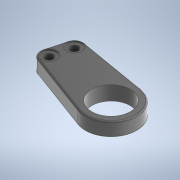
# Autodesk Inventor part: RearBumper
Saved by Autodesk Inventor 2020.4 (Build 244396000, 396)
## iProperties
Created: 2022-01-16
Part Number: RearBumper
Material: PC/ABS プラスチック
Document SubType Name: Modeling
Designer: Masato Kubotera
Density: 0.357273 g/cm^3
Appearance: 滑らか - 黒
Author: Masato Kubotera
Autodesk Inventor part; units mm, degrees
ref_plane "YZ Plane" through (0, 0, 0) normal (1, 0, 0) x (0, 1, 0)
ref_plane "XZ Plane" through (0, 0, 0) normal (0, 1, 0) x (-1, 0, 0)
ref_plane "XY Plane" through (0, 0, 0) normal (0, 0, 1) x (1, 0, 0)
derived "Trunk_basis.ipt"
sketch "スケッチ1" plane through (0, 0, 0) normal (0, 1, 0) x (-1, 0, 0)
  line L0 (0, 22) -> (0, -142.9) construction
  circle A0 centre (5, 0) radius 10.5 construction
  line L1 (-7, 16) -> (36, 16) construction
  line L2 (36, 16) -> (36, -16) construction
  line L3 (36, -16) -> (-7, -16) construction
  line L4 (-7, -16) -> (-7, 16) construction
  line L5 (-7, 16) -> (36, -16) construction
  line L6 (36, 16) -> (-7, -16) construction
  line L7 (33, 13.5) -> (6, 13.5) construction
  line L8 (6, 13.5) -> (6, -13.5) construction
  line L9 (6, -13.5) -> (33, -13.5) construction
  line L10 (33, -13.5) -> (33, 13.5) construction
  line L11 (33, 13.5) -> (6, -13.5) construction
  line L12 (6, 13.5) -> (33, -13.5) construction
  line L13 (-7, 0) -> (36, 0) construction
  arc A1 (5, 16) -> (-7, 10.583) centre (5, 0) ccw construction
  line L14 (34.5651, -16.05) -> (5, -16.05)
  line L15 (5, 16.05) -> (34.5651, 16.05)
  line L16 (36.05, 14.5651) -> (36.05, -14.5651)
  line L17 (36.05, -16.05) -> (-7.05, 16.05) construction
  line L18 (-7.05, -16.05) -> (36.05, 16.05) construction
  arc A2 (5, 16.05) -> (-6.5314, 11.1638) centre (5, 0) ccw
  arc A3 (-6.5314, 11.1638) -> (-7.05, 9.8372) centre (-6.0721, 10.2196) ccw
  arc A4 (36.05, 14.5651) -> (34.5651, 16.05) centre (35.3075, 15.3075) ccw
  circle A5 centre (6, 13.5) radius 1.35
  line L19 (19.5, 13.5) -> (19.5, -13.5) construction
  circle A6 centre (33, 13.5) radius 1.35
  line L20 (-12, 22) -> (-17, 17)
  line L21 (-17, 17) -> (-17, -16)
  line L22 (-17, -16) -> (-28.5, -27.5)
  line L23 (-28.5, -27.5) -> (-28.5, -103)
  line L24 (54.5, -22.5) -> (54.5, 17)
  line L25 (54.5, 17) -> (49.5, 22)
  line L26 (49.5, 22) -> (-12, 22)
  line L27 (-35.5597, -116.5529) -> (-28.5, -142.9)
  line L28 (-16, -139) -> (-16, -94) construction
  line L29 (-7.5, -140.4849) -> (-7.5, -142.9)
  line L30 (-7.5, -142.9) -> (7.5, -142.9)
  line L31 (7.5, -140.4849) -> (7.5, -142.9)
  arc A7 (-7.5, -140.4849) -> (-8.9849, -139) centre (-8.2425, -139.7425) ccw
  line L32 (-17.5, -138.9955) -> (-17.5, -133) construction
  line L33 (-19, -133) -> (-16, -133) construction
  line L34 (-19, -133) -> (-19, -139) construction
  line L35 (-16, -133) -> (-16, -139) construction
  line L36 (-12, 22) -> (-7, 22) construction
  line L37 (-7, 22) -> (-7, -22) construction
  line L38 (-7, -22) -> (-12, -22) construction
  line L39 (-12, -22) -> (-12, 22) construction
  line L40 (-12, 22) -> (-7, -22) construction
  line L41 (-7, 22) -> (-12, -22) construction
  line L42 (-9.5, 22) -> (-9.5, -22) construction
  line L43 (-7, 0) -> (-12, 0) construction
  circle A8 centre (-9.5, 17.75) radius 1.6
  line L44 (-12, 10) -> (-9.5, 10) construction
  line L45 (-9.5, 10) -> (-9.5, -10) construction
  line L46 (-9.5, -10) -> (-12, -10) construction
  line L47 (-12, -10) -> (-12, 10) construction
  line L48 (-12, 10) -> (-9.5, -10) construction
  line L49 (-9.5, 10) -> (-12, -10) construction
  line L50 (-9.45, 10.05) -> (-12.05, 10.05)
  line L51 (-12.05, 7.95) -> (-12.05, -7.95)
  line L52 (-12.05, -10.05) -> (-9.45, -10.05)
  line L53 (-9.45, -7.95) -> (-9.45, 7.95)
  line L54 (-9.45, 10.05) -> (-12.05, -10.05) construction
  line L55 (-12.05, 10.05) -> (-9.45, -10.05) construction
  arc A9 (-12.05, 10.05) -> (-12.05, 7.95) centre (-12.05, 9) ccw
  line L56 (-10.75, 10) -> (-10.75, -10) construction
  arc A10 (-9.45, 7.95) -> (-9.45, 10.05) centre (-9.45, 9) ccw
  circle A11 centre (-9.5, -17.75) radius 1.6
  arc A12 (-12.05, -7.95) -> (-12.05, -10.05) centre (-12.05, -9) ccw
  arc A13 (-9.45, -10.05) -> (-9.45, -7.95) centre (-9.45, -9) ccw
  line L57 (36, 14.4) -> (44.5, 14.4) construction
  line L58 (44.5, 14.4) -> (44.5, -14.4) construction
  line L59 (36, -14.4) -> (44.5, -14.4) construction
  line L60 (46.95, 7.95) -> (46.95, -7.95)
  line L61 (49.5, 0) -> (44.5, 0) construction
  line L62 (44.5, 22) -> (49.5, 22) construction
  line L63 (49.55, -7.95) -> (49.55, 7.95)
  line L64 (48.25, 10) -> (48.25, -10) construction
  line L65 (49.5, 10) -> (47, -10) construction
  line L66 (49.5, -10) -> (47, -10) construction
  line L67 (49.5, 10) -> (49.5, -10) construction
  line L68 (47, 10) -> (49.5, -10) construction
  line L69 (46.95, -10.05) -> (49.55, -10.05)
  line L70 (46.95, 10.05) -> (49.55, -10.05) construction
  line L71 (49.55, 10.05) -> (46.95, -10.05) construction
  line L72 (49.5, -22) -> (44.5, -22) construction
  line L73 (44.5, 22) -> (49.5, -22) construction
  line L74 (49.5, 22) -> (49.5, -22) construction
  line L75 (49.5, 22) -> (44.5, -22) construction
  line L76 (47, 22) -> (47, -22) construction
  line L77 (44.5, -22) -> (44.5, 22) construction
  circle A14 centre (47, -17.75) radius 1.6
  arc A15 (49.55, -10.05) -> (49.55, -7.95) centre (49.55, -9) ccw
  line L78 (47, -10) -> (47, 10) construction
  arc A16 (46.95, -7.95) -> (46.95, -10.05) centre (46.95, -9) ccw
  arc A17 (46.95, 10.05) -> (46.95, 7.95) centre (46.95, 9) ccw
  arc A18 (49.55, 7.95) -> (49.55, 10.05) centre (49.55, 9) ccw
  line L79 (47, 10) -> (49.5, 10) construction
  line L80 (49.55, 10.05) -> (46.95, 10.05)
  circle A19 centre (47, 17.75) radius 1.6
  circle A20 centre (5, 0) radius 16 construction
  arc A21 (-6.5314, -11.1638) -> (5, -16.05) centre (5, 0) ccw
  arc A22 (-7.05, -9.8372) -> (-6.5314, -11.1638) centre (-6.0721, -10.2196) ccw
  arc A23 (34.5651, -16.05) -> (36.05, -14.5651) centre (35.3075, -15.3075) ccw
  line L81 (-7.05, -9.8372) -> (-7.05, 9.8372)
  line L82 (17.5, -138.9955) -> (17.5, -133) construction
  line L83 (19, -133) -> (19, -139) construction
  line L84 (16, -133) -> (16, -139) construction
  line L85 (19, -133) -> (16, -133) construction
  circle A24 centre (6, -13.5) radius 1.35
  circle A25 centre (33, -13.5) radius 1.35
  line L86 (-25.5, -142.9) -> (-7.5, -142.9) construction
  line L87 (25.5, -142.9) -> (7.5, -142.9) construction
  line L88 (-23.5, -22.5) -> (54.5, -22.5) construction
  line L89 (54.5, -22.5) -> (54.5, -103)
  circle A26 centre (-13.5, -55) radius 1.75
  line L90 (-16.5, -59) -> (42.5, -59)
  line L91 (44.5, -61) -> (44.5, -88)
  line L92 (42.5, -90) -> (-16.5, -90)
  line L93 (-18.5, -88) -> (-18.5, -61)
  line L94 (-18.5, -59) -> (44.5, -90) construction
  line L95 (44.5, -59) -> (-18.5, -90) construction
  line L96 (-16.5, -27.5) -> (42.5, -27.5)
  line L97 (44.5, -29.5) -> (44.5, -49)
  line L98 (42.5, -51) -> (-16.5, -51)
  line L99 (-18.5, -49) -> (-18.5, -29.5)
  line L100 (-18.5, -27.5) -> (44.5, -51) construction
  line L101 (44.5, -27.5) -> (-18.5, -51) construction
  line L102 (-23.5, -108) -> (-28.5, -103)
  circle A27 centre (-20.5415, -102) radius 1.6
  line L103 (-25.7227, -96) -> (25.7227, -96)
  line L104 (25.7227, -96) -> (34.9603, -112)
  line L105 (35.5597, -116.5529) -> (28.5, -142.9)
  line L106 (-25.7227, -96) -> (-34.9603, -112)
  line L107 (54.5, -103) -> (49.5, -108)
  arc A28 (-16.5, -27.5) -> (-18.5, -29.5) centre (-16.5, -29.5) ccw
  arc A29 (-18.5, -49) -> (-16.5, -51) centre (-16.5, -49) ccw
  arc A30 (42.5, -51) -> (44.5, -49) centre (42.5, -49) ccw
  arc A31 (44.5, -29.5) -> (42.5, -27.5) centre (42.5, -29.5) ccw
  arc A32 (-16.5, -59) -> (-18.5, -61) centre (-16.5, -61) ccw
  arc A33 (-18.5, -88) -> (-16.5, -90) centre (-16.5, -88) ccw
  arc A34 (42.5, -90) -> (44.5, -88) centre (42.5, -88) ccw
  arc A35 (44.5, -61) -> (42.5, -59) centre (42.5, -61) ccw
  line L108 (-23.5, -108) -> (49.5, -108)
  line L109 (-25.5, -139) -> (-25.5, -142.9)
  line L110 (-25.5, -142.9) -> (-28.5, -142.9)
  line L111 (-17.9813, -99.3843) -> (-16.9961, -101.0907)
  line L112 (-16.9961, -102.9093) -> (-17.9813, -104.6157)
  line L113 (-19.5563, -105.525) -> (-21.5266, -105.525)
  line L114 (-23.1016, -104.6157) -> (-24.0868, -102.9093)
  line L115 (-24.0868, -101.0907) -> (-23.1016, -99.3843)
  line L116 (-21.5266, -98.475) -> (-19.5563, -98.475)
  line L117 (-16, -94) -> (16, -94) construction
  arc A36 (-24.0868, -101.0907) -> (-24.0868, -102.9093) centre (-23.5618, -102) ccw
  arc A37 (-23.1016, -104.6157) -> (-21.5266, -105.525) centre (-22.0516, -104.6157) ccw
  arc A38 (-19.5563, -105.525) -> (-17.9813, -104.6157) centre (-19.0313, -104.6157) ccw
  arc A39 (-16.9961, -102.9093) -> (-16.9961, -101.0907) centre (-17.5211, -102) ccw
  arc A40 (-17.9813, -99.3843) -> (-19.5563, -98.475) centre (-19.0313, -99.3843) ccw
  arc A41 (-21.5266, -98.475) -> (-23.1016, -99.3843) centre (-22.0516, -99.3843) ccw
  line L118 (16, -139) -> (16, -94) construction
  line L119 (16, -94) -> (-16, -94) construction
  line L120 (-25.5, -139) -> (-8.9849, -139)
  line L121 (25.5, -142.9) -> (28.5, -142.9)
  arc A42 (8.9849, -139) -> (7.5, -140.4849) centre (8.2425, -139.7425) ccw
  circle A43 centre (29.7641, -115) radius 1.25
  line L122 (33.4891, -124.2803) -> (21.898, -121.1745) construction
  line L123 (29.7641, -115) -> (25.623, -130.4548) construction
  circle A44 centre (29.7641, -115) radius 6 construction
  circle A45 centre (-20.5415, -102) radius 6 construction
  line L124 (1.9319, -109.4824) -> (7.5588, -130.4824)
  line L125 (5.6269, -133) -> (-5.6269, -133)
  line L126 (5.3151, -110.5176) -> (10.942, -131.5176)
  line L127 (12.8739, -133) -> (17.1947, -133)
  line L128 (19.1266, -131.5176) -> (24.7535, -110.5176)
  line L129 (22.8217, -108) -> (7.2469, -108)
  circle A46 centre (25.623, -130.4548) radius 1.25
  circle A47 centre (25.623, -130.4548) radius 6 construction
  line L130 (-1.9319, -109.4824) -> (-7.5588, -130.4824)
  arc A48 (1.9319, -109.4824) -> (-1.9319, -109.4824) centre (0, -110) ccw
  arc A49 (-7.5588, -130.4824) -> (-5.6269, -133) centre (-5.6269, -131) ccw
  arc A50 (5.6269, -133) -> (7.5588, -130.4824) centre (5.6269, -131) ccw
  arc A51 (7.2469, -108) -> (5.3151, -110.5176) centre (7.2469, -110) ccw
  arc A52 (24.7535, -110.5176) -> (22.8217, -108) centre (22.8217, -110) ccw
  arc A53 (17.1947, -133) -> (19.1266, -131.5176) centre (17.1947, -131) ccw
  arc A54 (10.942, -131.5176) -> (12.8739, -133) centre (12.8739, -131) ccw
  arc A55 (-5.3151, -110.5176) -> (-7.2469, -108) centre (-7.2469, -110) ccw
  line L131 (-22.8217, -108) -> (-7.2469, -108)
  line L132 (-5.3151, -110.5176) -> (-10.942, -131.5176)
  arc A56 (-22.8217, -108) -> (-24.7535, -110.5176) centre (-22.8217, -110) ccw
  line L133 (-19.1266, -131.5176) -> (-24.7535, -110.5176)
  arc A57 (-19.1266, -131.5176) -> (-17.1947, -133) centre (-17.1947, -131) ccw
  line L134 (-12.8739, -133) -> (-17.1947, -133)
  arc A58 (-12.8739, -133) -> (-10.942, -131.5176) centre (-12.8739, -131) ccw
  circle A59 centre (-29.7641, -115) radius 1.25
  circle A60 centre (-25.623, -130.4548) radius 1.25
  arc A61 (35.5597, -116.5529) -> (34.9603, -112) centre (29.7641, -115) ccw
  arc A62 (-34.9603, -112) -> (-35.5597, -116.5529) centre (-29.7641, -115) ccw
  arc A63 (-24.0151, -139) -> (-25.5, -140.4849) centre (-24.7575, -139.7425) ccw
  line L135 (25.5, -139) -> (25.5, -142.9)
  arc A64 (25.5, -140.4849) -> (24.0151, -139) centre (24.7575, -139.7425) ccw
  line L136 (25.5, -139) -> (8.9849, -139)
  line L137 (21.5266, -98.475) -> (19.5563, -98.475)
  line L138 (16.9961, -102.9093) -> (17.9813, -104.6157)
  arc A65 (21.5266, -105.525) -> (23.1016, -104.6157) centre (22.0516, -104.6157) ccw
  circle A66 centre (20.5415, -102) radius 1.6
  line L139 (24.0868, -101.0907) -> (23.1016, -99.3843)
  arc A67 (24.0868, -102.9093) -> (24.0868, -101.0907) centre (23.5618, -102) ccw
  line L140 (23.1016, -104.6157) -> (24.0868, -102.9093)
  arc A68 (23.1016, -99.3843) -> (21.5266, -98.475) centre (22.0516, -99.3843) ccw
  line L141 (19.5563, -105.525) -> (21.5266, -105.525)
  arc A69 (19.5563, -98.475) -> (17.9813, -99.3843) centre (19.0313, -99.3843) ccw
  arc A70 (17.9813, -104.6157) -> (19.5563, -105.525) centre (19.0313, -104.6157) ccw
  line L142 (17.9813, -99.3843) -> (16.9961, -101.0907)
  arc A71 (16.9961, -101.0907) -> (16.9961, -102.9093) centre (17.5211, -102) ccw
  line L143 (16, -139) -> (16, -94) construction
  circle A72 centre (20.5415, -102) radius 6 construction
  arc A73 (29.5045, -117.5445) -> (31.2612, -117.0738) centre (30.247, -116.802) ccw construction
  line L144 (31.8379, -116.4971) -> (31.2612, -117.0738) construction
  line L145 (29.5045, -117.5445) -> (28.7167, -117.3334) construction
  arc A74 (27.4307, -116.0474) -> (28.7167, -117.3334) centre (28.4449, -116.3192) ccw construction
  line L146 (27.4307, -116.0474) -> (27.2196, -115.2596) construction
  line L147 (27.6903, -113.5029) -> (28.267, -112.9262) construction
  arc A75 (30.0237, -112.4555) -> (28.267, -112.9262) centre (29.2813, -113.198) ccw construction
  arc A76 (27.6903, -113.5029) -> (27.2196, -115.2596) centre (27.9621, -114.5171) ccw construction
  line L148 (30.0237, -112.4555) -> (30.8116, -112.6666) construction
  arc A77 (31.8379, -116.4971) -> (32.3086, -114.7404) centre (31.5662, -115.4829) ccw construction
  arc A78 (32.0975, -113.9526) -> (30.8116, -112.6666) centre (31.0833, -113.6808) ccw construction
  line L149 (32.0975, -113.9526) -> (32.3086, -114.7404) construction
  point P0 (0, 0)
  point P1 (14.5, 0)
  point P2 (19.5, 0)
  point P3 (-7.05, 10.6019)
  point P4 (19.5, 0)
  point P5 (-9.5, 0)
  point P6 (-10.75, 0)
  point P7 (36.05, 14.4)
  point P8 (36.05, -14.4)
  point P9 (48.25, 0)
  point P10 (47, 0)
  point P11 (13, -74.5)
  point P12 (13, -39.25)
  point P13 (-18.5063, -98.475)
  point P14 (-16.4711, -102)
  point P15 (-18.5063, -105.525)
  point P16 (-22.5766, -105.525)
  point P17 (-22.5766, -98.475)
  point P18 (-24.6118, -102)
  point P19 (-22.5766, -105.525)
  point P20 (-18.5063, -105.525)
  point P21 (-16.4711, -102)
  point P22 (-18.5063, -98.475)
  point P23 (-22.5766, -98.475)
  point P24 (27.6936, -122.7274)
  point P25 (0, -102.2726)
  point P26 (0, -133)
  point P27 (-7.5, -139)
  point P28 (-22.5766, -98.475)
  point P29 (18.5063, -98.475)
  point P30 (18.5063, -98.475)
  point P31 (22.5766, -105.525)
  point P32 (22.5766, -105.525)
  point P33 (24.6118, -102)
  point P34 (22.5766, -98.475)
  point P35 (22.5766, -98.475)
  point P36 (22.5766, -98.475)
  point P37 (18.5063, -105.525)
  point P38 (16.4711, -102)
  point P39 (16.4711, -102)
  point P40 (18.5063, -105.525)
  point P41 (29.7641, -115)
  point P42 (29.7641, -115)
  point P43 (30.5187, -117.8163)
  point P44 (30.5187, -117.8163)
  point P45 (27.7025, -117.0617)
  point P46 (27.7025, -117.0617)
  point P47 (31.8258, -112.9383)
  point P48 (26.9479, -114.2454)
  point P49 (29.0095, -112.1837)
  point P50 (29.0095, -112.1837)
  point P51 (31.8258, -112.9383)
  point P52 (29.0095, -112.1837)
  point P53 (32.5804, -115.7546)
sketch "スケッチ2" plane through (0, 0, 0) normal (0, 1, 0) x (-1, 0, 0)
  circle A0 centre (29.7641, -115) radius 1.25 projected
  circle A1 centre (25.623, -130.4548) radius 1.25 projected
  circle A2 centre (29.7641, -115) radius 3.25
  arc A3 (30.9394, -108.0994) -> (23.0026, -113.1883) centre (29.7641, -115) ccw
  line L0 (30.9394, -108.0994) -> (83.3579, -117.0268)
  circle A4 centre (80, -136.7429) radius 15
  circle A5 centre (80, -136.7429) radius 20
  line L1 (33.4891, -124.2803) -> (21.898, -121.1745) construction
  circle A6 centre (25.623, -130.4548) radius 3.25
  arc A7 (18.8615, -128.6431) -> (23.1905, -137.0186) centre (25.623, -130.4548) ccw
  line L2 (23.1905, -137.0186) -> (73.0499, -155.4964)
  line L3 (0, 22) -> (0, -142.9) construction
  line L4 (23.0026, -113.1883) -> (18.8615, -128.6431)
  circle A8 centre (29.7641, -115) radius 6
  circle A9 centre (25.623, -130.4548) radius 6
  point P0 (0, 0)
  point P1 (73.0499, -155.4964)
  dimension "d4" = 40
  dimension "d1" = 6.5
  dimension "d2" = 7
  dimension "d3" = 30
  dimension "d5" = 80
  dimension "d6" = 12
  constraints: 7 centre point, 6 end point, 6 symmetric about line, 5 coincident, 4 point on circle, 2 tangent, 1 point on line, 7 other
  measures "d1" diameter of A2
  measures "d2" radius of A3
  measures "d3" diameter of A4
  measures "d5" horizontal distance of A4.centre L3.end
  measures "d6" diameter of A8
extrude "押し出し1" add sketch "スケッチ2" along normal blind 11 contours L0 A5 L2 A7 L4 A3 | A5
extrude "押し出し2" add sketch "スケッチ2" along normal blind 10 contours A8 | A9
extrude "押し出し3" cut sketch "スケッチ2" along normal blind 1 contours A8 | A9
fillet "フィレット1" radius 1 12 edges at (-99.3185, 11, -141.9193) (-57.1486, 11, -112.5631) (-25.9858, 11, -109.1073) (-20.9321, 11, -120.9157) (-19.4045, 11, -133.6689) (-48.1202, 11, -146.2575) (-99.3185, 0, -141.9193) (-57.1486, 0, -112.5631) (-25.9858, 0, -109.1073) (-20.9321, 0, -120.9157) (-19.4045, 0, -133.6689) (-48.1202, 0, -146.2575)
